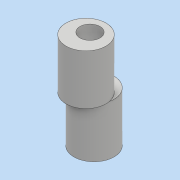
# Autodesk Inventor part: offset 6id 12- od 9mm
Saved by Autodesk Inventor 2020.2 (Build 242310000, 310)
## iProperties
Created: 2017-01-01
Part Number: offset 6id 12- od 9mm
Material: Allgemein
Document SubType Name: Modeling
Designer: paulg
Density: 1 g/cm^3
Appearance: Vorgabe
Author: paulg
Autodesk Inventor part; units mm, degrees
ref_plane "YZ Plane" through (0, 0, 0) normal (1, 0, 0) x (0, 1, 0)
ref_plane "XZ Plane" through (0, 0, 0) normal (0, 1, 0) x (-1, 0, 0)
ref_plane "XY Plane" through (0, 0, 0) normal (0, 0, 1) x (1, 0, 0)
sketch "Sketch1" plane through (0, 0, 0) normal (0, 0, 1) x (1, 0, 0)
  circle A0 centre (0, 1) radius 5
  line L0 (0, 0) -> (0, 1) construction
  dimension "d0" = 1
  dimension "d1" = 10
  constraints: 2 end point, 1 centre point, 1 vertical
  measures "d0" distance of L0.start L0.end
  measures "d1" diameter of A0
extrude "Extrusion1" add sketch "Sketch1" along normal blind 12.5
sketch "Sketch2" plane through (0, 1, 12.5) normal (0, 0, 1) x (1, 0, 0)
  circle A0 centre (0, -2) radius 5
  line L0 (0, -1) -> (0, -2) construction
  dimension "d4" = 1
  dimension "d5" = 10
  constraints: 2 end point, 1 centre point, 1 vertical
  measures "d4" distance of L0.start L0.end
  measures "d5" diameter of A0
extrude "Extrusion2" add sketch "Sketch2" along normal blind 12.5
sketch "Sketch3" plane through (0, -1, 25) normal (0, 0, 1) x (1, 0, 0)
  circle A0 centre (0, 1) radius 2.5
  dimension "d8" = 5
  constraints: 1 centre point, 1 coincident
  measures "d8" diameter of A0
extrude "Extrusion3" cut sketch "Sketch3" against normal through all
equation "\"d5\" = d1"
body "Solid1"
